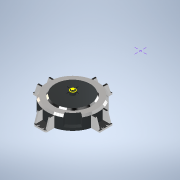
# Autodesk Inventor part: base
Saved by Autodesk Inventor 2022 (Build 260153000, 153)
## iProperties
Created: 2023-11-29
Part Number: base
Material: Generic
Document SubType Name: Modeling
Designer: harshidd
Density: 1 g/cm^3
Appearance: Iron Gray
Author: harshidd
Autodesk Inventor part; units mm, degrees
ref_plane "YZ Plane" through (0, 0, 0) normal (1, 0, 0) x (0, 1, 0)
sketch "Sketch1" plane through (0, 0, 0) normal (0, 1, 0) x (-1, 0, 0)
  circle A0 centre (0, 0) radius 150
  dimension "d0" = 300
  constraints: 1 centre point, 1 coincident
  measures "d0" diameter of A0
extrude "Extrusion1" add sketch "Sketch1" along normal blind 75
chamfer "Chamfer1" distance 10 angle 45 1 edges at (150, 75, 0)
sketch "Sketch2" plane through (0, 0, 0) normal (0, -1, 0) x (1, 0, 0)
  line L0 (-195.3522, -37.0505) -> (-145.3522, -37.0505)
  line L1 (-145.1202, 37.9491) -> (-195.1222, 37.9491)
  line L2 (-195.1222, 37.9491) -> (-195.3522, -37.0505)
  circle A0 centre (0, 0) radius 150 projected
  line L3 (-195.3522, -37.0505) -> (-116.2547, 27.9738) construction
  line L4 (-116.2547, -27.9738) -> (-195.1222, 37.9491) construction
  arc A1 (-145.1202, 37.9491) -> (-145.3522, -37.0505) centre (0, 0) ccw
  point P0 (-149.9998, 0.2327)
  dimension "d9" = 75
  dimension "d10" = 50
  constraints: 10 end point, 6 point on circle, 2 point on line, 1 centre point, 1 horizontal, 1 parallel
  measures "d9" distance of L1.end L0.start
  measures "d10" distance of L0.end L0.start
extrude "Extrusion2" add sketch "Sketch2" against normal blind 10 contours L2 L1 A0 L0
chamfer "Chamfer2" distance 7 angle 45 2 edges at (-195.1222, 5, 37.9491) (-195.3522, 5, -37.0505)
sketch "Sketch3" plane through (-145.1202, 0, 37.9491) normal (0, 0, 1) x (1, 0, 0)
  line L0 (-43.002, 10) -> (0, 10) projected
  line L1 (-43.002, 10) -> (0, 10)
  line L2 (0, 10) -> (0, 65)
  line L3 (295.1202, 65) -> (-4.8798, 65) projected
  line L4 (0, 65) -> (-25.002, 65)
  line L5 (-25.002, 65) -> (-43.002, 10)
  point P0 (145.1202, 0)
  point P1 (-0.232, 10)
  dimension "d16" = 18
  constraints: 8 end point, 2 point on line, 1 collinear, 1 perpendicular
  measures "d16" horizontal distance of L4.end L0.start
extrude "Extrusion3" add sketch "Sketch3" against normal blind 9
sketch "Sketch4" plane through (0, 10, 0) normal (0, 1, 0) x (1, 0, 0)
  line L0 (-145.3522, 37.0505) -> (-188.3522, 37.0505) projected
  line L1 (-188.3522, 37.0505) -> (-188.3522, -49.5813)
  line L2 (-188.1222, -37.9491) -> (-188.1222, -28.9491) projected
  line L3 (-188.3522, 0) -> (-188.3522, -14.25)
  line L4 (-188.3522, -8.25) -> (-183.156, -11.25)
  line L5 (-183.156, -11.25) -> (-183.156, -17.25)
  line L6 (-183.156, -17.25) -> (-188.3522, -20.25)
  line L7 (-188.3522, -20.25) -> (-193.5483, -17.25)
  line L8 (-193.5483, -17.25) -> (-193.5483, -11.25)
  line L9 (-193.5483, -11.25) -> (-188.3522, -8.25)
  point P0 (0, 0)
  dimension "d19" = 14.25
  dimension "d20" = 6
  constraints: 16 end point, 3 point on line, 1 coincident, 1 parallel, 13 other
  measures "d19" distance of L3.start L3.end
  measures "d20" distance of L4.end L5.end
extrude "Extrusion4" add sketch "Sketch4" along normal blind 3.5
sketch "Sketch5" plane through (0, 10, 0) normal (0, 1, 0) x (1, 0, 0)
  point P0 (0, 0)
ref_plane "Work Plane1" through (-188.1222, 0, 0.4491) normal (0, 0, 1) x (1, 0, 0)
mirror "Mirror1" about plane through (-188.1222, 0, 0.4491) normal (0, 0, 1) of "Extrusion3", "Extrusion4"
pattern_circular "Circular Pattern1" count 4 over 360 about axis through (0, 0, 0) along (0, 1, 0) of "Extrusion3", "Extrusion4", "Mirror1", "Extrusion2"
sketch "Sketch6" plane through (0, 75, 0) normal (0, 1, 0) x (1, 0, 0)
  line L0 (-37.0505, -195.3522) -> (37.9491, -195.1222) projected
  line L1 (-110.0762, -63.5525) -> (-129.9038, -75)
  line L2 (-63.2147, -110.2705) -> (-74.6013, -130.1332)
  arc A0 (-110.0762, -63.5525) -> (-63.2147, -110.2705) centre (0, 0) ccw
  arc A1 (-129.9038, -75) -> (-74.6013, -130.1332) centre (0, 0) ccw
  constraints: 4 end point, 4 point on circle, 2 centre point, 2 coincident
extrude "Extrusion5" cut sketch "Sketch6" against normal blind 60
sketch "Sketch7" plane through (0, 75, 0) normal (0, 1, 0) x (1, 0, 0)
  circle A0 centre (0, 0) radius 110
  dimension "d31" = 220
  constraints: 1 centre point, 1 coincident
  measures "d31" diameter of A0
ref_plane "Work Plane2" through (0, 82, 0) normal (0, 1, 0) x (1, 0, 0)
sketch "Sketch8" plane through (0, 82, 0) normal (0, 1, 0) x (1, 0, 0)
  circle A0 centre (0, 0) radius 102.5
  dimension "d33" = 205
  constraints: 1 centre point, 1 coincident
  measures "d33" diameter of A0
loft "Loft1" add profiles "Sketch7", "Sketch8"
sketch "Sketch9" plane through (0, 82, 0) normal (0, 1, 0) x (1, 0, 0)
  circle A0 centre (0, 0) radius 15
  dimension "d38" = 30
  constraints: 1 centre point, 1 coincident
  measures "d38" diameter of A0
extrude "Extrusion6" add sketch "Sketch9" along normal blind 20
sketch "Sketch10" plane through (0, 102, 0) normal (0, 1, 0) x (1, 0, 0)
  circle A0 centre (0, 0) radius 15 projected
  point P0 (398.7645, 0)
  point P1 (398.7645, 0)
  constraints: 2 coincident
body "Solid1"
